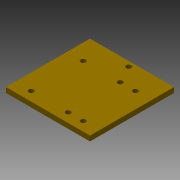
# Autodesk Inventor part: X Rail
Saved by Autodesk Inventor 2013 SP2 (Build 170200200, 200)
## iProperties
Created: 2017-01-25
Part Number: X Rail
Material: Generic
Document SubType Name: Modeling
Designer: Herman de Vries
Density: 1 g/cm^3
Mass: 83.894 g
Surface Area: 597.307 cm^2
Volume: 83.894 cm^3
Author: Herman de Vries
Autodesk Inventor part; units mm, degrees
ref_plane "YZ Plane" through (0, 0, 0) normal (1, 0, 0) x (0, 1, 0)
ref_plane "XZ Plane" through (0, 0, 0) normal (0, 1, 0) x (-1, 0, 0)
ref_plane "XY Plane" through (0, 0, 0) normal (0, 0, 1) x (1, 0, 0)
sketch "Sketch1" plane through (0, 0, 0) normal (1, 0, 0) x (0, 1, 0)
  line L0 (0, 0) -> (50, 0)
  line L1 (50, 0) -> (50, 3)
  line L2 (50, 3) -> (0, 3)
  line L3 (0, 3) -> (0, 0)
  dimension "d0" = 50
  dimension "d1" = 3
  constraints: 8 end point, 2 parallel, 1 horizontal, 1 perpendicular
  measures "d0" distance of L2.end L1.end
  measures "d1" distance of L1.end L0.end
extrude "Extrusion1" add sketch "Sketch1" along normal blind 50
sketch "Sketch2" plane through (0, 0, 3) normal (0, 0, 1) x (1, 0, 0)
  line L0 (0, 0) -> (50, 0) projected
  line L1 (0, 50) -> (50, 50) projected
  line L2 (0, 50) -> (0, 0) projected
  line L3 (50, 50) -> (50, 0) projected
  line L4 (9.5, 36.5) -> (40.5, 36.5) construction
  line L5 (40.5, 36.5) -> (40.5, 5.5) construction
  line L6 (40.5, 5.5) -> (9.5, 5.5) construction
  line L7 (9.5, 5.5) -> (9.5, 36.5) construction
  circle A0 centre (9.5, 36.5) radius 1.5
  circle A1 centre (40.5, 36.5) radius 1.5
  circle A2 centre (40.5, 5.5) radius 1.5
  circle A3 centre (9.5, 5.5) radius 1.5
  circle A4 centre (56.8804, 53.3963) radius 1.5
  circle A5 centre (26, 30) radius 1.5
  circle A6 centre (26, 3) radius 1.5
  circle A7 centre (31.5, 47) radius 1.5
  circle A8 centre (31.5, 3) radius 1.5
  point P0 (50, 25)
  point P1 (9.5, 21)
  point P2 (0, 25)
  point P3 (25, 36.5)
  point P4 (25, 50)
  point P5 (13.7786, -2.6691)
  dimension "d12" = 31
  dimension "d13" = 31
  dimension "d15" = 3
  dimension "d16" = 3
  dimension "d17" = 3
  dimension "d18" = 3
  dimension "d19" = 3
  dimension "d21" = 3
  dimension "d22" = 3
  dimension "d23" = 20
  dimension "d24" = 3
  dimension "d26" = 5.5
  dimension "d27" = 26
  dimension "d28" = 3
  dimension "d29" = 3
  dimension "d31" = 3
  dimension "d32" = 3
  dimension "d33" = 9
  constraints: 9 centre point, 8 end point, 5 midpoint, 4 coincident, 3 vertical alignment, 2 parallel, 1 horizontal, 1 perpendicular
  measures "d12" distance of L5.end L6.end
  measures "d13" distance of L4.end L5.end
  measures "d15" diameter of A0
  measures "d16" diameter of A1
  measures "d17" diameter of A2
  measures "d18" diameter of A3
  measures "d19" diameter of A4
  measures "d21" diameter of A5
  measures "d22" diameter of A6
  measures "d23" distance from line of L1 A5.centre
  measures "d24" distance from line of L0 A6.centre
  measures "d26" distance between parallel lines of L0 L6
  measures "d27" distance from line of A6.centre L2
  measures "d28" diameter of A7
  measures "d29" diameter of A8
  measures "d31" distance from line of L1 A7.centre
  measures "d32" distance from line of L0 A8.centre
  measures "d33" horizontal distance of L5.end A8.centre
extrude "Extrusion2" cut sketch "Sketch2" against normal blind 10 contours A0 | A1 | A2 | A3 | A4 | A5 | A7 | A8
equation "\"d12\" = d13"
body "Solid1"
